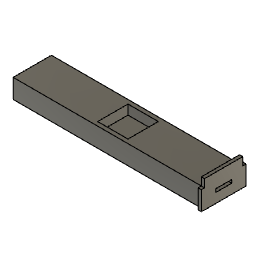
final project v4 (Autodesk Fusion 360 design; units mm, degrees)
Autodesk Fusion 360 part; units mm, degrees
sketch "草图1" plane through (0, 0, 0) normal (0, 0, 1) x (1, 0, 0)
sketch "草图2" plane through (0, 0, 0) normal (0, 0, 1) x (1, 0, 0)
  line L0 (-60, 15) -> (60, 15)
  line L1 (60, 15) -> (60, -10)
  line L2 (60, -10) -> (-60, -10)
  line L3 (-60, -10) -> (-60, 15)
  constraint horizontal L0
  constraint vertical L1
  constraint horizontal L2
  constraint vertical L3
sketch "草图3" plane through (0, 0, 0) normal (0, 0, 1) x (1, 0, 0)
  line L0 (-59.8985, 12.4694) -> (60.1015, 12.4694)
  line L1 (60.1015, 12.4694) -> (60.1015, -11.5306)
  line L2 (60.1015, -11.5306) -> (-59.8985, -11.5306)
  line L3 (-59.8985, -11.5306) -> (-59.8985, 12.4694)
  dimension "d5" = 120
  dimension "d6" = 24
  constraint horizontal L0
  constraint vertical L1
  constraint horizontal L2
  constraint vertical L3
  measures "d5" distance of L0.start L0.end
  measures "d6" distance of L0.start L2.end
sketch "草图4" plane through (0, 0, 0) normal (0, 0, 1) x (1, 0, 0)
  line L0 (-9.3981, 9.9691) -> (9.6019, 9.9691)
  line L1 (9.6019, 9.9691) -> (9.6019, -9.0309)
  line L2 (9.6019, -9.0309) -> (-9.3981, -9.0309)
  line L3 (-9.3981, -9.0309) -> (-9.3981, 9.9691)
  dimension "d9" = 19
  dimension "d10" = 19
  constraint horizontal L0
  constraint vertical L1
  constraint horizontal L2
  constraint vertical L3
  measures "d9" distance of L0.start L0.end
  measures "d10" distance of L0.start L2.end
extrude "拉伸2" add sketch "草图3" along normal mid plane 12
extrude "拉伸3" cut sketch "草图4" along normal blind 6
sketch "草图5" plane through (0, 0, 6) normal (0, 0, 1) x (-1, 0, 0)
  line L0 (9.3981, 9.0309) -> (9.3981, -9.9691)
  line L1 (9.3981, -9.9691) -> (-9.6019, -9.9691)
  line L2 (-9.6019, -9.9691) -> (-9.6019, 9.0309)
  line L3 (-9.6019, 9.0309) -> (9.3981, 9.0309)
  line L4 (59.8985, 11.5306) -> (-60.1015, 11.5306)
  line L5 (-60.1015, 11.5306) -> (-60.1015, -12.4694)
  line L6 (-60.1015, -12.4694) -> (59.8985, -12.4694)
  line L7 (59.8985, -12.4694) -> (59.8985, 11.5306)
  line L8 (-9.6019, -5.4698, -6) -> (-60.1672, -5.4698, -6)
  line L9 (-60.1672, -5.4698, -6) -> (-60.1672, 4.5302, -6)
  line L10 (-60.1672, 4.5302, -6) -> (-9.6019, 4.5302, -6)
  line L11 (-9.6019, 4.5302, -6) -> (-9.6019, -5.4698, -6)
extrude "拉伸4" cut sketch "草图5" along normal blind 3 contours L8 L9 L10 L11 in plane through (0, 0, 0) normal (0, 0, 1)
sketch "草图6" plane through (0, 0, 0) normal (0, 0, 1) x (1, 0, 0)
  line L0 (58.1015, 12.4694) -> (60.1015, 12.4694)
  line L1 (60.1015, 12.4694) -> (60.1015, -11.5306)
  line L2 (60.1015, -11.5306) -> (58.1015, -11.5306)
  line L3 (58.1015, -11.5306) -> (58.1015, 12.4694)
  point P0 (60.1015, 12.4694)
  constraint coincident P0 L0.end
extrude "拉伸5" add sketch "草图6" along normal blind 9 from surface at 2
sketch "草图7" plane through (0, 0, 0) normal (0, 0, 1) x (1, 0, 0)
  line L0 (58.1015, 14.4694) -> (60.1015, 14.4694)
  line L1 (60.1015, 14.4694) -> (60.1015, 12.4694)
  line L2 (60.1015, 12.4694) -> (58.1015, 12.4694)
  line L3 (58.1015, 12.4694) -> (58.1015, 14.4694)
  point P0 (60.1015, 12.4694)
  dimension "d23" = 2
  constraint horizontal L0
  constraint vertical L1
  constraint horizontal L2
  constraint vertical L3
  constraint coincident P0 L1.end
  measures "d23" distance of L0.start L0.end
extrude "拉伸6" add sketch "草图7" along normal mid plane 12
sketch "草图8" plane through (0, 0, 0) normal (0, 0, 1) x (1, 0, 0)
  line L0 (58.1015, -11.5306) -> (60.1015, -11.5306)
  line L1 (60.1015, -11.5306) -> (60.1015, -13.5306)
  line L2 (60.1015, -13.5306) -> (58.1015, -13.5306)
  line L3 (58.1015, -13.5306) -> (58.1015, -11.5306)
  point P0 (60.1015, -11.5306)
  dimension "d26" = 2
  dimension "d27" = 2
  constraint horizontal L0
  constraint vertical L1
  constraint horizontal L2
  constraint vertical L3
  constraint coincident P0 L0.end
  measures "d26" distance of L0.start P0
  measures "d27" distance of L0.start L2.end
extrude "拉伸7" add sketch "草图8" along normal mid plane 12
